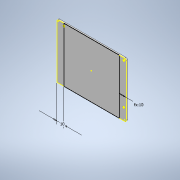
# Autodesk Inventor part: NanoHolder
Saved by Autodesk Inventor 2022 (Build 260153000, 153)
## iProperties
Created: 2021-04-23
Part Number: NanoHolder
Material: Generic
Document SubType Name: Modeling
Designer: Viktor
Density: 1 g/cm^3
Appearance: Default
Author: Viktor
Autodesk Inventor part; units mm, degrees
ref_plane "YZ Plane" through (0, 0, 0) normal (1, 0, 0) x (0, 1, 0)
ref_plane "XZ Plane" through (0, 0, 0) normal (0, 1, 0) x (-1, 0, 0)
ref_plane "XY Plane" through (0, 0, 0) normal (0, 0, 1) x (1, 0, 0)
sketch "Sketch1" plane through (0, 0, 0) normal (0, 0, 1) x (1, 0, 0)
  line L0 (-50, -39.5) -> (50, -39.5)
  line L1 (50, -39.5) -> (50, 39.5)
  line L2 (50, 39.5) -> (-50, 39.5)
  line L3 (-50, 39.5) -> (-50, -39.5)
  line L4 (-50, -39.5) -> (50, 39.5) construction
  line L5 (50, -39.5) -> (-50, 39.5) construction
  point P0 (0, 0)
  dimension "d0" = 100
  dimension "d1" = 79
  constraints: 12 end point, 2 midpoint, 2 parallel, 1 horizontal, 1 perpendicular
  measures "d0" distance of L1.end L2.end
  measures "d1" distance of L0.end L1.end
extrude "Extrusion1" add sketch "Sketch1" along normal blind 2
sketch "Sketch3" plane through (0, 0, 2) normal (0, 0, 1) x (1, 0, 0)
  circle A0 centre (-40, 36) radius 1.25
  circle A1 centre (46.5, 36) radius 1.25
  circle A2 centre (46.5, -22.7) radius 1.25
  line L0 (-50, 39.5) -> (-50, -39.5) projected
  line L1 (50, 39.5) -> (-50, 39.5) projected
  line L2 (50, -39.5) -> (50, 39.5) projected
  line L3 (-50, -39.5) -> (50, -39.5) projected
  point P0 (0, 0)
  dimension "d6" = 2.5
  dimension "d7" = 2.5
  dimension "d8" = 2.5
  dimension "d9" = 10
  dimension "d10" = 3.5
  dimension "d11" = 3.5
  dimension "d12" = 3.5
  dimension "d13" = 3.5
  dimension "d14" = 16.8
  constraints: 3 centre point
  measures "d6" diameter of A0
  measures "d7" diameter of A1
  measures "d8" diameter of A2
  measures "d9" distance from line of L0 A0.centre
  measures "d10" distance from line of L1 A0.centre
  measures "d11" distance from line of L2 A1.centre
  measures "d12" distance from line of L1 A1.centre
  measures "d13" distance from line of L2 A2.centre
  measures "d14" distance from line of L3 A2.centre
extrude "Extrusion2" cut sketch "Sketch3" against normal blind 2 contours A0 | A1 | A2
fillet "Fillet1" radius 2 3 edges at (50, -39.5, 1) (50, 39.5, 1) (-50, 39.5, 1)
sketch "Sketch4" plane through (0, 0, 2) normal (0, 0, 1) x (1, 0, 0)
  arc A0 (-48, 39.5) -> (-50, 37.5) centre (-48, 37.5) ccw projected
  line L0 (-50, 37.5) -> (-50, -39.5) projected
  line L1 (-50, -39.5) -> (48, -39.5) projected
  arc A1 (48, -39.5) -> (50, -37.5) centre (48, -37.5) ccw projected
  line L2 (50, -37.5) -> (50, 37.5) projected
  arc A2 (50, 37.5) -> (48, 39.5) centre (48, 37.5) ccw projected
  line L3 (48, 39.5) -> (-48, 39.5) projected
  circle A3 centre (-40, 36) radius 1.25 projected
  circle A4 centre (46.5, 36) radius 1.25 projected
  circle A5 centre (46.5, -22.7) radius 1.25 projected
  line L4 (-50, -39.5) -> (48, -39.5) projected
  line L5 (48, 39.5) -> (-48, 39.5) projected
  line L6 (-40, -39.5) -> (40, -39.5)
  line L7 (40, -39.5) -> (40, 39.5)
  line L8 (40, 39.5) -> (-40, 39.5)
  line L9 (-40, 39.5) -> (-40, -39.5)
  point P0 (0, 0)
  dimension "d18" = 10
  dimension "d19" = 10
  constraints: 8 end point, 2 parallel, 2 point on line, 1 horizontal, 1 perpendicular
  measures "d18" distance between parallel lines of L0 L9
  measures "d19" distance between parallel lines of L2 L7
equation "\"d7\" = d6"
equation "\"d8\" = d6"
equation "\"d11\" = d10"
equation "\"d12\" = d11"
equation "\"d13\" = d12"
equation "\"d19\" = d18"
body "Solid1"
